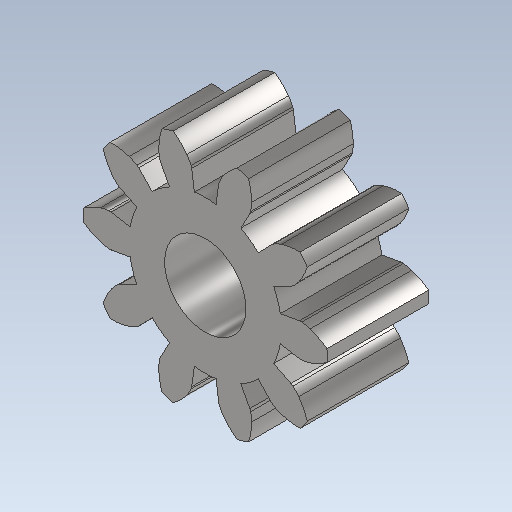
# Autodesk Inventor part: m1歯数10焼結ギア5td4
Saved by Autodesk Inventor 2020.2 (Build 242310000, 310)
## iProperties
Created: 2020-02-29
Part Number: m1歯数10焼結ギア5td4
Material: 鋼、炭素鋼
Document SubType Name: Modeling
Designer: aoyam
Density: 7.85 g/cm^3
Appearance: 半つや出し
Author: aoyam
Autodesk Inventor part; units mm, degrees
ref_plane "YZ Plane" through (0, 0, 0) normal (1, 0, 0) x (0, 1, 0)
ref_plane "XZ Plane" through (0, 0, 0) normal (0, 1, 0) x (-1, 0, 0)
ref_plane "XY Plane" through (0, 0, 0) normal (0, 0, 1) x (1, 0, 0)
sketch "スケッチ1" plane through (0, 0, 0) normal (0, 0, 1) x (1, 0, 0)
  arc A0 (-0.1284, 7.9518) -> (-0.1636, 7.8356) centre (0.4243, 7.7211) ccw
  arc A1 (0.0762, 8.3168) -> (-0.1284, 7.9518) centre (1.4214, 7.3228) ccw
  arc A2 (0.7431, 8.9748) -> (0.0762, 8.3168) centre (2.4847, 6.5424) ccw
  arc A3 (-1.4951, 7.8356) -> (-1.5303, 7.9518) centre (-2.0831, 7.7211) ccw
  arc A4 (-1.5303, 7.9518) -> (-1.7349, 8.3168) centre (-3.0802, 7.3228) ccw
  arc A5 (-1.7349, 8.3168) -> (-2.4019, 8.9748) centre (-4.1434, 6.5424) ccw
  arc A6 (-0.298, 6.8967) -> (-1.3607, 6.8967) centre (-0.8294, 3.1845) ccw
  arc A7 (-2.4019, 8.9748) -> (-2.9606, 8.7932) centre (-0.8294, 3.1845) ccw
  line L0 (-0.298, 6.8967) -> (-0.1636, 7.8356)
  line L1 (-1.3607, 6.8967) -> (-1.4951, 7.8356)
  line L2 (-3.4412, 5.8754) -> (-4.1018, 6.556)
  arc A8 (-4.1018, 6.556) -> (-4.1986, 6.6293) centre (-4.5102, 6.1177) ccw
  arc A9 (-4.1986, 6.6293) -> (-4.5787, 6.8044) centre (-5.0828, 5.2095) ccw
  arc A10 (-4.5787, 6.8044) -> (-5.505, 6.9446) centre (-5.4842, 3.9532) ccw
  arc A11 (-5.505, 6.9446) -> (-5.8503, 6.4694) centre (-0.8294, 3.1845) ccw
  arc A12 (-2.5815, 6.5) -> (-3.4412, 5.8754) centre (-0.8294, 3.1845) ccw
  line L3 (-2.5815, 6.5) -> (-3.0246, 7.3386)
  arc A13 (-3.0645, 7.4533) -> (-3.0246, 7.3386) centre (-2.4816, 7.5916) ccw
  arc A14 (-3.1135, 7.8689) -> (-3.0645, 7.4533) centre (-1.4409, 7.8555) ccw
  arc A15 (-2.9606, 8.7932) -> (-3.1135, 7.8689) centre (-0.122, 7.8491) ccw
  line L4 (-4.5241, 3.8263) -> (-5.4585, 3.9886)
  arc A16 (-5.4585, 3.9886) -> (-5.58, 3.9911) centre (-5.5313, 3.394) ccw
  arc A17 (-5.58, 3.9911) -> (-5.9903, 3.9093) centre (-5.4607, 2.3226) ccw
  arc A18 (-5.9903, 3.9093) -> (-6.8222, 3.4782) centre (-5.047, 1.0703) ccw
  arc A19 (-6.8222, 3.4782) -> (-6.8222, 2.8908) centre (-0.8294, 3.1845) ccw
  arc A20 (-4.1957, 4.837) -> (-4.5241, 3.8263) centre (-0.8294, 3.1845) ccw
  line L5 (-4.1957, 4.837) -> (-5.0471, 5.2549)
  arc A21 (-5.1468, 5.3243) -> (-5.0471, 5.2549) centre (-4.7565, 5.7787) ccw
  arc A22 (-5.4306, 5.6317) -> (-5.1468, 5.3243) centre (-4.0696, 6.604) ccw
  arc A23 (-5.8503, 6.4694) -> (-5.4306, 5.6317) centre (-2.9988, 7.374) ccw
  line L6 (-4.1957, 1.532) -> (-5.0471, 1.1141)
  arc A24 (-5.0471, 1.1141) -> (-5.1468, 1.0447) centre (-4.7565, 0.5903) ccw
  arc A25 (-5.1468, 1.0447) -> (-5.4306, 0.7373) centre (-4.0696, -0.235) ccw
  arc A26 (-5.4306, 0.7373) -> (-5.8503, -0.1003) centre (-2.9988, -1.005) ccw
  arc A27 (-5.8503, -0.1003) -> (-5.505, -0.5756) centre (-0.8294, 3.1845) ccw
  arc A28 (-4.5241, 2.5427) -> (-4.1957, 1.532) centre (-0.8294, 3.1845) ccw
  line L7 (-4.5241, 2.5427) -> (-5.4585, 2.3804)
  arc A29 (-5.58, 2.378) -> (-5.4585, 2.3804) centre (-5.5313, 2.975) ccw
  arc A30 (-5.9903, 2.4598) -> (-5.58, 2.378) centre (-5.4607, 4.0464) ccw
  arc A31 (-6.8222, 2.8908) -> (-5.9903, 2.4598) centre (-5.047, 5.2987) ccw
  line L8 (-2.5815, -0.131) -> (-3.0246, -0.9696)
  arc A32 (-3.0246, -0.9696) -> (-3.0645, -1.0843) centre (-2.4816, -1.2226) ccw
  arc A33 (-3.0645, -1.0843) -> (-3.1135, -1.4999) centre (-1.4409, -1.4864) ccw
  arc A34 (-3.1135, -1.4999) -> (-2.9606, -2.4242) centre (-0.122, -1.48) ccw
  arc A35 (-2.9606, -2.4242) -> (-2.4019, -2.6058) centre (-0.8294, 3.1845) ccw
  arc A36 (-3.4412, 0.4936) -> (-2.5815, -0.131) centre (-0.8294, 3.1845) ccw
  line L9 (-3.4412, 0.4936) -> (-4.1018, -0.187)
  arc A37 (-4.1986, -0.2603) -> (-4.1018, -0.187) centre (-4.5102, 0.2513) ccw
  arc A38 (-4.5787, -0.4353) -> (-4.1986, -0.2603) centre (-5.0828, 1.1596) ccw
  arc A39 (-5.505, -0.5756) -> (-4.5787, -0.4353) centre (-5.4842, 2.4159) ccw
  line L10 (-0.298, -0.5277) -> (-0.1636, -1.4665)
  arc A40 (-0.1636, -1.4665) -> (-0.1284, -1.5828) centre (0.4243, -1.352) ccw
  arc A41 (-0.1284, -1.5828) -> (0.0762, -1.9478) centre (1.4214, -0.9538) ccw
  arc A42 (0.0762, -1.9478) -> (0.7431, -2.6058) centre (2.4847, -0.1734) ccw
  arc A43 (0.7431, -2.6058) -> (1.3019, -2.4242) centre (-0.8294, 3.1845) ccw
  arc A44 (-1.3607, -0.5277) -> (-0.298, -0.5277) centre (-0.8294, 3.1845) ccw
  line L11 (-1.3607, -0.5277) -> (-1.4951, -1.4665)
  arc A45 (-1.5303, -1.5828) -> (-1.4951, -1.4665) centre (-2.0831, -1.352) ccw
  arc A46 (-1.7349, -1.9478) -> (-1.5303, -1.5828) centre (-3.0802, -0.9538) ccw
  arc A47 (-2.4019, -2.6058) -> (-1.7349, -1.9478) centre (-4.1434, -0.1734) ccw
  line L12 (1.7825, 0.4936) -> (2.4431, -0.187)
  arc A48 (2.4431, -0.187) -> (2.5398, -0.2603) centre (2.8514, 0.2513) ccw
  arc A49 (2.5398, -0.2603) -> (2.9199, -0.4353) centre (3.424, 1.1596) ccw
  arc A50 (2.9199, -0.4353) -> (3.8462, -0.5756) centre (3.8255, 2.4159) ccw
  arc A51 (3.8462, -0.5756) -> (4.1916, -0.1003) centre (-0.8294, 3.1845) ccw
  arc A52 (0.9227, -0.131) -> (1.7825, 0.4936) centre (-0.8294, 3.1845) ccw
  line L13 (0.9227, -0.131) -> (1.3658, -0.9696)
  arc A53 (1.4057, -1.0843) -> (1.3658, -0.9696) centre (0.8229, -1.2226) ccw
  arc A54 (1.4547, -1.4999) -> (1.4057, -1.0843) centre (-0.2179, -1.4864) ccw
  arc A55 (1.3019, -2.4242) -> (1.4547, -1.4999) centre (-1.5368, -1.48) ccw
  line L14 (2.8653, 2.5427) -> (3.7998, 2.3804)
  arc A56 (3.7998, 2.3804) -> (3.9212, 2.378) centre (3.8726, 2.975) ccw
  arc A57 (3.9212, 2.378) -> (4.3315, 2.4598) centre (3.8019, 4.0464) ccw
  arc A58 (4.3315, 2.4598) -> (5.1634, 2.8908) centre (3.3883, 5.2987) ccw
  arc A59 (5.1634, 2.8908) -> (5.1634, 3.4782) centre (-0.8294, 3.1845) ccw
  arc A60 (2.5369, 1.532) -> (2.8653, 2.5427) centre (-0.8294, 3.1845) ccw
  line L15 (2.5369, 1.532) -> (3.3883, 1.1141)
  arc A61 (3.488, 1.0447) -> (3.3883, 1.1141) centre (3.0977, 0.5903) ccw
  arc A62 (3.7719, 0.7373) -> (3.488, 1.0447) centre (2.4108, -0.235) ccw
  arc A63 (4.1916, -0.1003) -> (3.7719, 0.7373) centre (1.3401, -1.005) ccw
  line L16 (2.5369, 4.837) -> (3.3883, 5.2549)
  arc A64 (3.3883, 5.2549) -> (3.488, 5.3243) centre (3.0977, 5.7787) ccw
  arc A65 (3.488, 5.3243) -> (3.7719, 5.6317) centre (2.4108, 6.604) ccw
  arc A66 (3.7719, 5.6317) -> (4.1916, 6.4694) centre (1.3401, 7.374) ccw
  arc A67 (4.1916, 6.4694) -> (3.8462, 6.9446) centre (-0.8294, 3.1845) ccw
  arc A68 (2.8653, 3.8263) -> (2.5369, 4.837) centre (-0.8294, 3.1845) ccw
  line L17 (2.8653, 3.8263) -> (3.7998, 3.9886)
  arc A69 (3.9212, 3.9911) -> (3.7998, 3.9886) centre (3.8726, 3.394) ccw
  arc A70 (4.3315, 3.9093) -> (3.9212, 3.9911) centre (3.8019, 2.3226) ccw
  arc A71 (5.1634, 3.4782) -> (4.3315, 3.9093) centre (3.3883, 1.0703) ccw
  line L18 (0.9227, 6.5) -> (1.3658, 7.3386)
  arc A72 (1.3658, 7.3386) -> (1.4057, 7.4533) centre (0.8229, 7.5916) ccw
  arc A73 (1.4057, 7.4533) -> (1.4547, 7.8689) centre (-0.2179, 7.8555) ccw
  arc A74 (1.4547, 7.8689) -> (1.3019, 8.7932) centre (-1.5368, 7.8491) ccw
  arc A75 (1.3019, 8.7932) -> (0.7431, 8.9748) centre (-0.8294, 3.1845) ccw
  arc A76 (1.7825, 5.8754) -> (0.9227, 6.5) centre (-0.8294, 3.1845) ccw
  line L19 (1.7825, 5.8754) -> (2.4431, 6.556)
  arc A77 (2.5398, 6.6293) -> (2.4431, 6.556) centre (2.8514, 6.1177) ccw
  arc A78 (2.9199, 6.8044) -> (2.5398, 6.6293) centre (3.424, 5.2095) ccw
  arc A79 (3.8462, 6.9446) -> (2.9199, 6.8044) centre (3.8255, 3.9532) ccw
  circle A80 centre (-0.8294, 3.1845) radius 2
  point P0 (0, 0)
  point P1 (-0.1319, -1.5742)
  point P2 (0.073, -1.9435)
  point P3 (0.7431, -2.6058)
  point P4 (1.3019, -2.4242)
  point P5 (1.4547, -1.4946)
  point P6 (1.4035, -1.0753)
  point P7 (2.4431, -0.187)
  point P8 (2.532, -0.2554)
  point P9 (2.9149, -0.4337)
  point P10 (3.8462, -0.5756)
  point P11 (4.1916, -0.1003)
  point P12 (3.7688, 0.7416)
  point P13 (3.4809, 1.0507)
  point P14 (3.3883, 1.1141)
  point P15 (2.5369, 1.532)
  point P16 (3.912, 2.3773)
  point P17 (4.3265, 2.4581)
  point P18 (5.1634, 2.8908)
  point P19 (5.1634, 3.4782)
  point P20 (4.3265, 3.9109)
  point P21 (3.912, 3.9917)
  point P22 (2.8653, 3.8263)
  point P23 (2.5369, 4.837)
  point P24 (3.4809, 5.3184)
  point P25 (3.7688, 5.6274)
  point P26 (4.1916, 6.4694)
  point P27 (3.8462, 6.9446)
  point P28 (2.9149, 6.8028)
  point P29 (2.532, 6.6245)
  point P30 (1.3658, 7.3386)
  point P31 (1.4035, 7.4444)
  point P32 (1.4547, 7.8636)
  point P33 (1.3019, 8.7932)
  point P34 (0.7431, 8.9748)
  point P35 (0.073, 8.3125)
  point P36 (-0.1319, 7.9433)
  point P37 (-0.1636, 7.8356)
  point P38 (-0.298, 6.8967)
  point P39 (-1.3607, 6.8967)
  point P40 (-1.4951, 7.8356)
  point P41 (-1.5269, 7.9432)
  point P42 (-1.7318, 8.3125)
  point P43 (-2.4019, 8.9748)
  point P44 (-2.9606, 8.7932)
  point P45 (-3.1135, 7.8636)
  point P46 (-3.0623, 7.4444)
  point P47 (-3.0246, 7.3386)
  point P48 (-2.5815, 6.5)
  point P49 (-3.4412, 5.8754)
  point P50 (-4.1018, 6.556)
  point P51 (-4.1907, 6.6245)
  point P52 (-4.5736, 6.8028)
  point P53 (-5.505, 6.9446)
  point P54 (-5.8503, 6.4694)
  point P55 (-5.4276, 5.6274)
  point P56 (-5.1397, 5.3184)
  point P57 (-5.5707, 3.9917)
  point P58 (-5.9853, 3.9109)
  point P59 (-6.8222, 3.4782)
  point P60 (-6.8222, 2.8908)
  point P61 (-5.9853, 2.4581)
  point P62 (-5.5707, 2.3773)
  point P63 (-5.1397, 1.0507)
  point P64 (-5.4276, 0.7416)
  point P65 (-5.8503, -0.1003)
  point P66 (-5.505, -0.5756)
  point P67 (-4.5736, -0.4337)
  point P68 (-4.1907, -0.2554)
  point P69 (-3.0623, -1.0753)
  point P70 (-3.1135, -1.4946)
  point P71 (-2.9606, -2.4242)
  point P72 (-2.4019, -2.6058)
  point P73 (-1.7318, -1.9435)
  point P74 (-1.5268, -1.5742)
  point P75 (-1.4951, -1.4665)
  dimension "d2" = 360
  dimension "d4" = 4
  constraints: 160 point on circle, 81 centre point, 40 end point, 3 coincident, 379 other
  measures "d4" diameter of A80
extrude "押し出し1" add sketch "スケッチ1" along normal blind 5
